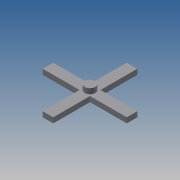
# Autodesk Inventor part: vertex
Saved by Autodesk Inventor 2014 SP1 (Build 180222100, 222)
## iProperties
Created: 2014-08-28
Part Number: vertex
Material: Generic
Document SubType Name: Modeling
Designer: Dave
Density: 1 g/cm^3
Appearance: Default
Author: Dave
Autodesk Inventor part; units mm, degrees
ref_plane "YZ Plane" through (0, 0, 0) normal (1, 0, 0) x (0, 1, 0)
ref_plane "XZ Plane" through (0, 0, 0) normal (0, 1, 0) x (-1, 0, 0)
ref_plane "XY Plane" through (0, 0, 0) normal (0, 0, 1) x (1, 0, 0)
sketch "Sketch1" plane through (0, 0, 0) normal (0, 1, 0) x (-1, 0, 0)
  line L0 (193.99, 66.5128) -> (193.99, 91.9128)
  line L1 (-9.21, 91.9128) -> (-9.21, 66.5128)
  line L2 (79.69, 180.8128) -> (105.09, 180.8128)
  line L3 (105.09, -22.3872) -> (79.69, -22.3872)
  line L4 (92.39, 180.8128) -> (92.39, -22.3872) construction
  line L5 (92.39, 91.9128) -> (92.39, 66.5128) construction
  line L6 (79.69, 79.2128) -> (105.09, 79.2128) construction
  line L7 (-9.21, 79.2128) -> (193.99, 79.2128) construction
  line L8 (193.99, 91.9128) -> (105.09, 91.9128)
  line L9 (79.69, 91.9128) -> (-9.21, 91.9128)
  line L10 (79.69, -22.3872) -> (79.69, 66.5128)
  line L11 (79.69, 91.9128) -> (79.69, 180.8128)
  line L12 (-9.21, 66.5128) -> (79.69, 66.5128)
  line L13 (105.09, 66.5128) -> (193.99, 66.5128)
  line L14 (105.09, 180.8128) -> (105.09, 91.9128)
  line L15 (105.09, 66.5128) -> (105.09, -22.3872)
  point P0 (0, 0)
  point P1 (92.39, 79.2128)
  dimension "d0" = 203.2
  dimension "d1" = 25.4
  dimension "d2" = 25.4
  dimension "d3" = 203.2
  constraints: 32 end point, 10 parallel, 6 midpoint, 4 perpendicular, 3 horizontal, 3 point on line
  measures "d0" distance of L1.start L0.end
  measures "d1" distance of L0.end L0.start
  measures "d2" distance of L3.start L3.end
  measures "d3" distance of L2.end L3.start
extrude "Extrusion1" add sketch "Sketch1" along normal blind 12.7
sketch "Sketch2" plane through (0, 12.7, 0) normal (0, 1, 0) x (1, 0, 0)
  circle A0 centre (-92.39, -79.2128) radius 12.7
  point P0 (0, 0)
  dimension "d7" = 25.4
  constraints: 1 centre point
  measures "d7" diameter of A0
extrude "Extrusion2" add sketch "Sketch2" along normal blind 12.7
body "Solid1"
